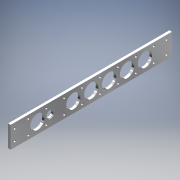
# Autodesk Inventor part: Outer Plate Module
Saved by Autodesk Inventor 2019.4 (Build 234330000, 330)
## iProperties
Created: 2020-01-01
Part Number: Outer Plate Module
Material: Aluminum 6061
Document SubType Name: Modeling
Designer: Mark
Mass: 353.145 g
Surface Area: 526.69 cm^2
Volume: 130.794 cm^3
Density: 2.7 g/cm^3
Appearance: Aluminum - Flat
Author: Mark
Autodesk Inventor part; units mm, degrees
ref_plane "YZ Plane" through (0, 0, 0) normal (1, 0, 0) x (0, 1, 0)
ref_plane "XZ Plane" through (0, 0, 0) normal (0, 1, 0) x (-1, 0, 0)
ref_plane "XY Plane" through (0, 0, 0) normal (0, 0, 1) x (1, 0, 0)
sketch "Sketch1" plane through (0, 0, 0) normal (1, 0, 0) x (0, 1, 0)
  circle A0 centre (0, 0) radius 9.5
  line L0 (-30, -110.28) -> (30, -110.28)
  line L1 (30, -110.28) -> (30, 110.28)
  line L2 (30, 110.28) -> (-30, 110.28)
  line L3 (-30, 110.28) -> (-30, -110.28)
  line L4 (-30, -110.28) -> (30, 110.28) construction
  line L5 (30, -110.28) -> (-30, 110.28) construction
  line L6 (30, -110.28) -> (-30, -110.28)
  line L7 (-30, -110.28) -> (-30, -339.72)
  line L8 (-30, -339.72) -> (30, -339.72)
  line L9 (30, -339.72) -> (30, -110.28)
  circle A1 centre (0, -311.7) radius 3.25
  dimension "d0" = 19
  dimension "d1" = 60
  dimension "d2" = 220.56
  dimension "d5" = 60
  dimension "d6" = 229.44
  dimension "d8" = 6.5
  dimension "d9" = 28.02
  dimension "d10" = 30
  constraints: 20 end point, 4 parallel, 2 centre point, 2 horizontal, 2 midpoint, 2 perpendicular, 1 coincident
  measures "d0" diameter of A0
  measures "d1" distance of L2.end L1.end
  measures "d2" distance of L1.end L0.end
  measures "d5" distance of L8.end L7.end
  measures "d6" distance of L7.end L6.end
  measures "d8" diameter of A1
  measures "d9" distance from line of L8 A1.centre
  measures "d10" distance from line of L7 A1.centre
extrude "Extrusion1" add sketch "Sketch1" along normal blind 7 contours L3 L2 L1 L0 | L0 L9 L8 L7 | A1
sketch "Sketch2" plane through (7, 0, 0) normal (-1, 0, 0) x (0, 0, 1)
  circle A0 centre (0, 0) radius 11
  dimension "d11" = 22
  constraints: 1 centre point, 1 coincident
  measures "d11" diameter of A0
extrude "Extrusion2" cut sketch "Sketch2" along normal blind 1.2
sketch "Sketch3" plane through (7, 0, 0) normal (1, 0, 0) x (0, 0, -1)
  circle A0 centre (-98.28, 15) radius 2.75
  circle A1 centre (-98.28, -15) radius 2.75
  circle A2 centre (324.72, 18) radius 2.75
  circle A3 centre (324.72, -18) radius 2.75
  line L0 (-110.28, -30) -> (339.72, -30) projected
  line L1 (339.72, 30) -> (-110.28, 30) projected
  line L2 (339.72, -30) -> (339.72, 30) projected
  line L3 (-110.28, 30) -> (-110.28, -30) projected
  line L4 (339.72, -30) -> (309.72, -30)
  line L5 (309.72, -30) -> (309.72, 30)
  line L6 (309.72, 30) -> (339.72, 30)
  line L7 (339.72, 30) -> (339.72, -30)
  line L8 (-110.28, -30) -> (-80.28, -30)
  line L9 (-80.28, -30) -> (-80.28, 30)
  line L10 (-80.28, 30) -> (-110.28, 30)
  line L11 (-110.28, 30) -> (-110.28, -30)
  circle A4 centre (-35.28, 0) radius 20
  line L12 (-60.28, -20) -> (-10.28, -20)
  line L13 (-10.28, -20) -> (-10.28, 20)
  line L14 (-10.28, 20) -> (-60.28, 20)
  line L15 (-60.28, 20) -> (-60.28, -20)
  line L16 (-60.28, -20) -> (-10.28, 20) construction
  line L17 (-10.28, -20) -> (-60.28, 20) construction
  circle A5 centre (-60.28, 20) radius 2.75
  circle A6 centre (-10.28, 20) radius 2.75
  circle A7 centre (-60.28, -20) radius 2.75
  circle A8 centre (-10.28, -20) radius 2.75
  circle A9 centre (-10.28, 20) radius 2.75
  circle A10 centre (-10.28, -20) radius 2.75
  circle A11 centre (14.72, 0) radius 20
  circle A12 centre (39.72, 20) radius 2.75
  circle A13 centre (39.72, -20) radius 2.75
  circle A14 centre (39.72, 20) radius 2.75
  circle A15 centre (39.72, -20) radius 2.75
  circle A16 centre (64.72, 0) radius 20
  circle A17 centre (89.72, 20) radius 2.75
  circle A18 centre (89.72, -20) radius 2.75
  circle A19 centre (89.72, 20) radius 2.75
  circle A20 centre (89.72, -20) radius 2.75
  circle A21 centre (114.72, 0) radius 20
  circle A22 centre (139.72, 20) radius 2.75
  circle A23 centre (139.72, -20) radius 2.75
  circle A24 centre (139.72, 20) radius 2.75
  circle A25 centre (139.72, -20) radius 2.75
  circle A26 centre (164.72, 0) radius 20
  circle A27 centre (189.72, 20) radius 2.75
  circle A28 centre (189.72, -20) radius 2.75
  circle A29 centre (189.72, 20) radius 2.75
  circle A30 centre (189.72, -20) radius 2.75
  circle A31 centre (214.72, 0) radius 20
  circle A32 centre (239.72, 20) radius 2.75
  circle A33 centre (239.72, -20) radius 2.75
  circle A34 centre (239.72, 20) radius 2.75
  circle A35 centre (239.72, -20) radius 2.75
  circle A36 centre (264.72, 0) radius 20
  circle A37 centre (289.72, 20) radius 2.75
  circle A38 centre (289.72, -20) radius 2.75
  circle A39 centre (289.72, 20) radius 2.75
  circle A40 centre (289.72, -20) radius 2.75
  circle A41 centre (314.72, 0) radius 20
  circle A42 centre (339.72, 20) radius 2.75
  circle A43 centre (339.72, -20) radius 2.75
  circle A44 centre (339.72, 20) radius 2.75
  circle A45 centre (339.72, -20) radius 2.75
  circle A46 centre (364.72, 0) radius 20
  circle A47 centre (389.72, 20) radius 2.75
  circle A48 centre (389.72, -20) radius 2.75
  circle A49 centre (389.72, 20) radius 2.75
  circle A50 centre (389.72, -20) radius 2.75
  circle A51 centre (414.72, 0) radius 20
  circle A52 centre (439.72, 20) radius 2.75
  circle A53 centre (439.72, -20) radius 2.75
  point P0 (0, 0)
  dimension "d14" = 5.5
  dimension "d15" = 5.5
  dimension "d16" = 5.5
  dimension "d17" = 5.5
  dimension "d18" = 12
  dimension "d19" = 12
  dimension "d20" = 15
  dimension "d21" = 15
  dimension "d22" = 15
  dimension "d23" = 12
  dimension "d24" = 12
  dimension "d25" = 15
  dimension "d26" = 30
  dimension "d27" = 30
  dimension "d28" = 60
  dimension "d29" = 40
  dimension "d30" = 50
  dimension "d31" = 40
  dimension "d32" = 75
  dimension "d33" = 10
  dimension "d34" = 5.5
  dimension "d35" = 5.5
  dimension "d36" = 5.5
  dimension "d37" = 5.5
  dimension "d40" = 50
  constraints: 54 centre point, 28 end point, 6 parallel, 4 coincident, 4 horizontal, 3 perpendicular, 2 midpoint, 1 point on line, 90 other
  measures "d14" diameter of A0
  measures "d15" diameter of A1
  measures "d16" diameter of A2
  measures "d17" diameter of A3
  measures "d18" distance from line of L0 A3.centre
  measures "d19" distance from line of L1 A2.centre
  measures "d20" distance from line of L2 A2.centre
  measures "d21" distance from line of L2 A3.centre
  measures "d22" distance from line of L1 A0.centre
  measures "d23" distance from line of L3 A0.centre
  measures "d24" distance from line of L3 A1.centre
  measures "d25" distance from line of L0 A1.centre
  measures "d26" distance of L5.end L6.end
  measures "d27" distance of L10.end L9.end
  measures "d28" distance of L9.end L8.end
  measures "d29" diameter of A4
  measures "d30" distance of L14.end L13.end
  measures "d31" distance of L13.end L12.end
  measures "d32" distance from line of L11 A4.centre
  measures "d33" distance between parallel lines of L0 L12
  measures "d34" diameter of A5
  measures "d35" diameter of A6
  measures "d36" diameter of A7
  measures "d37" diameter of A8
  measures "d40" distance of A5.centre A9.centre
extrude "Extrusion3" cut sketch "Sketch3" against normal blind 10 contours A0 | A1 | A2 A41 | A41 A2 | A41 A3 | A3 A41 | A4 | A6 L13 L14 | L14 L13 A6 | A5 L15 L14 | L14 L15 A5 | A7 L15 L12 | L12 L15 A7 | A8 L13 L12 | L12 L13 A8 | A12 | A13 | A16 | A17 | A18 | A21 | A22 | A23 | A26 | A27 | A28 | A31 | A32 | A33 | A36 | A37 | A38
body "Solid1"
